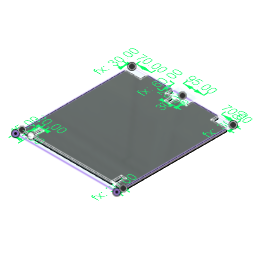
3030 Bottom MDF (Autodesk Fusion 360 design; units mm, degrees)
Autodesk Fusion 360 part; units mm, degrees
sketch "Sketch1" plane through (0, 0, 0) normal (0, 0, 1) x (1, 0, 0)
  line L0 (348.791, 124.3375) -> (818.791, 124.3375)
  line L1 (818.791, 124.3375) -> (818.791, -415.6625)
  line L2 (818.791, -415.6625) -> (348.791, -415.6625)
  line L3 (348.791, -415.6625) -> (348.791, 124.3375)
  dimension "d1701" = 470
  dimension "d1702" = 540
  constraint horizontal L0
  constraint vertical L1
  constraint horizontal L2
  constraint vertical L3
  measures "d1701" distance of L0.start L0.end
  measures "d1702" distance of L0.start L2.end
extrude "Extrude1" add sketch "Sketch1" along normal blind 12
sketch "Sketch6" plane through (0, 0, 12) normal (0, 0, 1) x (-1, 0, 0)
  line L0 (-348.791, 415.6625) -> (-818.791, 415.6625)
  line L1 (-818.791, 415.6625) -> (-818.791, -124.3375)
  line L2 (-818.791, -124.3375) -> (-348.791, -124.3375)
  line L3 (-348.791, -124.3375) -> (-348.791, 415.6625)
  line L4 (-348.791, -124.3375) -> (-418.791, -124.3375)
  line L5 (-418.791, -124.3375) -> (-418.791, -94.3375)
  line L6 (-418.791, -94.3375) -> (-348.791, -94.3375)
  line L7 (-348.791, -94.3375) -> (-348.791, -124.3375)
  line L8 (-818.791, -124.3375) -> (-748.791, -124.3375)
  line L9 (-748.791, -124.3375) -> (-748.791, -94.3375)
  line L10 (-748.791, -94.3375) -> (-818.791, -94.3375)
  line L11 (-818.791, -94.3375) -> (-818.791, -124.3375)
  line L12 (-631.291, -94.3375) -> (-536.291, -94.3375)
  line L13 (-536.291, -94.3375) -> (-536.291, -154.3375)
  line L14 (-536.291, -154.3375) -> (-631.291, -154.3375)
  line L15 (-631.291, -154.3375) -> (-631.291, -94.3375)
  line L16 (-631.291, -94.3375) -> (-536.291, -154.3375) construction
  line L17 (-536.291, -94.3375) -> (-631.291, -154.3375) construction
  line L18 (-583.791, -94.3375) -> (-583.791, -64.3375)
  line L19 (-583.791, -64.3375) -> (-563.791, -64.3375)
  line L20 (-563.791, -64.3375) -> (-563.791, -94.3375)
  line L21 (-348.791, 385.6625) -> (-818.791, 385.6625)
  line L22 (-382.791, 385.6625) -> (-402.791, 385.6625)
  line L23 (-402.791, 385.6625) -> (-402.791, 340.6625)
  line L24 (-402.791, 340.6625) -> (-382.791, 340.6625)
  line L25 (-382.791, 340.6625) -> (-382.791, 385.6625)
  line L26 (-392.791, 340.6625) -> (-392.791, 388.277) construction
  line L27 (-784.791, 340.6625) -> (-784.791, 385.6625)
  line L28 (-784.791, 385.6625) -> (-764.791, 385.6625)
  line L29 (-764.791, 385.6625) -> (-764.791, 340.6625)
  line L30 (-764.791, 340.6625) -> (-784.791, 340.6625)
  point P0 (-583.791, -124.3375)
  dimension "d8051" = 70
  dimension "d8052" = 30
  dimension "d8053" = 70
  dimension "d8054" = 30
  dimension "d8055" = 95
  dimension "d8056" = 60
  dimension "d8057" = 20
  dimension "d8058" = 30
  dimension "d8059" = 30
  dimension "d8060" = 20
  dimension "d8061" = 45
  dimension "d8063" = 44
  constraint horizontal L4
  constraint vertical L5
  constraint horizontal L6
  constraint vertical L7
  constraint coincident L2.end L3.start
  constraint horizontal L8
  constraint vertical L9
  constraint horizontal L10
  constraint vertical L11
  constraint coincident L1.end L2.start
  constraint horizontal L12
  constraint perpendicular L12 L13
  constraint parallel L12 L14
  constraint parallel L13 L15
  constraint coincident L16 P0
  constraint coincident L17 P0
  constraint midpoint L2 P0
  constraint midpoint L12 L18.start
  constraint perpendicular L12 L18
  constraint perpendicular L18 L19
  constraint coincident L12 L20.end
  constraint perpendicular L12 L20
  constraint coincident L3 L21.start
  constraint coincident L1 L21.end
  constraint perpendicular L1 L21
  constraint horizontal L22
  constraint vertical L23
  constraint horizontal L24
  constraint vertical L25
  constraint coincident L21 L22.start
  constraint midpoint L24 L26.start
  constraint perpendicular L24 L26
  constraint symmetric L18 L22.start L27.end
  constraint symmetric L18 L22.end L28.end
  constraint symmetric L18 L23.end L29.end
  constraint symmetric L18 L24.end L27.start
  measures "d8051" distance of L2.end L4.end
  measures "d8052" distance of L2.end L6.end
  measures "d8053" distance of L1.end L8.end
  measures "d8054" distance of L1.end L10.end
  measures "d8055" distance of L13.end L14.end
  measures "d8056" distance of L12.end L13.end
  measures "d8057" distance of L18.end L19.end
  measures "d8058" distance of L18.start L18.end
  measures "d8059" distance of L0.end L21.end
  measures "d8060" distance of L22.start L22.end
  measures "d8061" distance of L22.start L24.end
  measures "d8063" horizontal distance of L0.start L26.end
extrude "Extrude4" cut sketch "Sketch6" against normal up to surface (12 mm away) contours L0 L1 L3 L21 L22 L28 | L2 L3 L4 L5 L6 L7 | L21 L22 L23 L24 L25 | L1 L2 L8 L9 L10 L11 | L21 L27 L28 L29 L30 | L2 L12 L13 L15 | L12 L18 L19 L20
equation "d1701 = FrameSizeX"
equation "d1702 = FrameSizeY"
equation "d1703 = drybox_panel_thickness"
equation "d8052 = frameProfile"
equation "d8054 = frameProfile"
equation "d8056 = frameProfile * 2"
equation "d8059 = frameProfile"
equation "d8063 = 54 mm - 10 mm"
equation "FrameSizeX = 470 mm" comment "Frame Size Outer X"
equation "FrameSizeY = 540 mm" comment "Frame Size Outer Y"
equation "frameProfile = 30 mm"
equation "drybox_panel_thickness = 12 mm" comment "Drybox MDF thickness"
named bodies: "Bottom Hatch"
